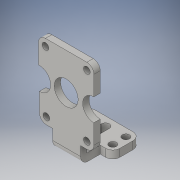
# Autodesk Inventor part: cwmotorholder
Saved by Autodesk Inventor 2016 (Build 200138000, 138)
## iProperties
Created: 2017-09-06
Part Number: cwmotorholder
Material: Generic
Document SubType Name: Modeling
Designer: student
Density: 1 g/cm^3
Appearance: Default
Author: student
Autodesk Inventor part; units mm, degrees
ref_plane "YZ Plane" through (0, 0, 0) normal (1, 0, 0) x (0, 1, 0)
ref_plane "XZ Plane" through (0, 0, 0) normal (0, 1, 0) x (-1, 0, 0)
ref_plane "XY Plane" through (0, 0, 0) normal (0, 0, 1) x (1, 0, 0)
sketch "Sketch1" plane through (0, 0, 0) normal (0, 0, 1) x (1, 0, 0)
  line L0 (8.2804, 14.6939) -> (-8.2804, 14.6939)
  circle A0 centre (0, 0) radius 4.7752
  line L1 (-7.8994, -15.0749) -> (-5.3848, -15.0749)
  line L2 (-5.3848, -15.0749) -> (-5.3848, -22.3393)
  line L3 (8.2804, -15.4559) -> (5.7658, -15.4559)
  line L4 (5.7658, -15.4559) -> (5.7658, -22.3393)
  line L5 (5.7658, -22.3393) -> (-5.3848, -22.3393)
  arc A1 (-10.6934, -4.8641) -> (-11.0744, 4.0859) centre (-10.6934, -0.381) ccw
  line L6 (-11.0744, 11.8999) -> (-11.0744, 4.0859)
  line L7 (-10.6934, -4.8641) -> (-10.6934, -12.2809)
  arc A2 (11.0744, 4.1021) -> (11.0744, -4.8641) centre (11.0744, -0.381) ccw
  line L8 (11.0744, -12.6619) -> (11.0744, -4.8641)
  line L9 (11.0744, 4.1021) -> (11.0744, 11.8999)
  arc A3 (-8.2804, 14.6939) -> (-11.0744, 11.8999) centre (-8.2804, 11.8999) ccw
  arc A4 (11.0744, 11.8999) -> (8.2804, 14.6939) centre (8.2804, 11.8999) ccw
  arc A5 (8.2804, -15.4559) -> (11.0744, -12.6619) centre (8.2804, -12.6619) ccw
  arc A6 (-10.6934, -12.2809) -> (-7.8994, -15.0749) centre (-7.8994, -12.2809) ccw
  circle A7 centre (-8.2804, 11.8999) radius 1.3335
  circle A8 centre (8.2804, 11.8999) radius 1.3335
  circle A9 centre (8.2804, -12.6619) radius 1.3335
  circle A10 centre (-7.8994, -12.2809) radius 1.3335
  point P0 (-10.6934, -15.0749)
  point P1 (11.0744, 14.6939)
  point P2 (11.0744, -15.4559)
  point P3 (-11.0744, 14.6939)
  dimension "d0" = 30.1498
  dimension "d1" = 22.1488
  dimension "d2" = 9.5504
  dimension "d3" = 5.3086
  dimension "d4" = 7.2644
  dimension "d5" = 5.3086
  dimension "d6" = 8.9662
  dimension "d7" = 8.9662
  dimension "d11" = 2.794
  dimension "d12" = 2.667
  dimension "d13" = 2.667
  dimension "d14" = 2.667
  dimension "d15" = 2.667
  constraints: 20 end point, 12 point on circle, 11 centre point, 8 point on line, 8 tangent, 5 coincident, 4 parallel, 3 equal radius, 3 perpendicular, 1 horizontal
  measures "d0" distance of point (11.074, -15.456) point (11.074, 14.694)
  measures "d1" distance of point (11.074, 14.694) point (-11.074, 14.694)
  measures "d2" diameter of A0
  measures "d3" distance of point (-10.693, -15.075) L1.end
  measures "d4" distance of L1.end L2.end
  measures "d5" distance of point (11.074, -15.456) L3.end
  measures "d6" diameter of A1
  measures "d7" diameter of A2
  measures "d11" radius of A3
  measures "d12" diameter of A7
  measures "d13" diameter of A8
  measures "d14" diameter of A9
  measures "d15" diameter of A10
extrude "Extrusion1" add sketch "Sketch1" along normal blind 2.54
fillet "Fillet1" radius 3.175 1 edges at (0.1905, -22.3393, 2.54)
sketch "Sketch2" plane through (0, 0, 0) normal (0, 0, -1) x (-1, 0, 0)
  line L0 (-5.7658, -19.2284) -> (5.3848, -19.2284) projected
  line L1 (-5.7658, -19.2284) -> (5.3848, -19.2284)
  line L2 (-5.7658, -22.3393) -> (-5.7658, -19.2284) projected
  line L3 (-5.7658, -19.2284) -> (-5.7658, -22.3393)
  line L4 (-5.7658, -22.3393) -> (5.3848, -22.3393) projected
  line L5 (-5.7658, -22.3393) -> (5.3848, -22.3393)
  line L6 (5.3848, -19.2284) -> (5.3848, -22.3393) projected
  line L7 (5.3848, -22.3393) -> (5.3848, -19.2284)
  point P0 (0, 0)
  constraints: 8 end point, 2 collinear, 1 horizontal, 1 vertical
extrude "Extrusion2" add sketch "Sketch2" along normal blind 5.334
sketch "Sketch6" plane through (-5.3848, -22.3393, 0) normal (0, -1, 0) x (1, 0, 0)
  line L0 (11.1506, -5.334) -> (13.3604, -5.334)
  line L1 (16.1544, -8.128) -> (16.1544, -13.335)
  line L2 (0, -5.334) -> (-2.2098, -5.334)
  line L3 (-5.0038, -8.128) -> (-5.0038, -13.335)
  line L4 (-1.8288, -16.51) -> (12.9794, -16.51)
  line L5 (0, -5.334) -> (11.1506, -5.334) projected
  line L6 (0, -5.334) -> (11.1506, -5.334)
  arc A0 (12.9794, -16.51) -> (16.1544, -13.335) centre (12.9794, -13.335) ccw
  arc A1 (-5.0038, -13.335) -> (-1.8288, -16.51) centre (-1.8288, -13.335) ccw
  arc A2 (16.1544, -8.128) -> (13.3604, -5.334) centre (13.3604, -8.128) ccw
  arc A3 (-2.2098, -5.334) -> (-5.0038, -8.128) centre (-2.2098, -8.128) ccw
  point P0 (5.3848, 0)
  point P1 (16.1544, -5.334)
  point P2 (16.1544, -16.51)
  point P3 (-5.0038, -5.334)
  point P4 (-5.0038, -16.51)
  dimension "d30" = 5.0038
  dimension "d32" = 5.0038
  dimension "d35" = 3.175
  dimension "d36" = 2.794
  constraints: 12 end point, 8 point on circle, 8 point on line, 8 tangent, 4 centre point, 3 perpendicular, 2 equal radius, 2 horizontal, 1 collinear
  measures "d30" distance of L0.start point (16.154, -5.334)
  measures "d32" distance of L2.start point (-5.004, -5.334)
  measures "d35" radius of A0
  measures "d36" radius of A2
extrude "Extrusion3" add sketch "Sketch6" against normal blind 3.1115
sketch "Sketch7" plane through (-5.3848, -19.2278, 0) normal (0, 1, 0) x (1, 0, 0)
  line L0 (0, 5.334) -> (11.1506, 5.334) projected
  line L1 (-1.8288, 16.51) -> (12.9794, 16.51) projected
  line L2 (3.9624, 12.9323) -> (3.9624, 3.1787)
  line L3 (7.1882, 3.1787) -> (7.1882, 12.9323)
  arc A0 (7.1882, 12.9323) -> (3.9624, 12.9323) centre (5.5753, 12.9323) ccw
  arc A1 (3.9624, 3.1787) -> (7.1882, 3.1787) centre (5.5753, 3.1787) ccw
  point P0 (5.3848, 0)
  point P1 (5.5753, 8.0555)
  dimension "d37" = 9.7536
  dimension "d38" = 3.2258
  constraints: 4 end point, 4 point on circle, 4 tangent, 2 centre point, 1 parallel
  measures "d37" distance of A0.centre A1.centre
  measures "d38" diameter of A1
extrude "Extrusion4" cut sketch "Sketch7" against normal blind 76.2
sketch "Sketch8" plane through (-5.3848, -19.2278, 0) normal (0, 1, 0) x (1, 0, 0)
  circle A0 centre (13.3829, 13.3417) radius 1.4351
  circle A1 centre (13.3829, 8.1013) radius 1.4355
  circle A2 centre (-2.1844, 8.1013) radius 1.4351
  circle A3 centre (-2.1844, 13.3417) radius 1.4351
  point P0 (5.3848, 0)
  dimension "d48" = 2.8702
  dimension "d49" = 2.8702
  dimension "d50" = 2.8702
  constraints: 4 centre point
  measures "d48" diameter of A0
  measures "d49" diameter of A2
  measures "d50" diameter of A3
extrude "Extrusion5" cut sketch "Sketch8" against normal blind 76.2
body "Solid1"
